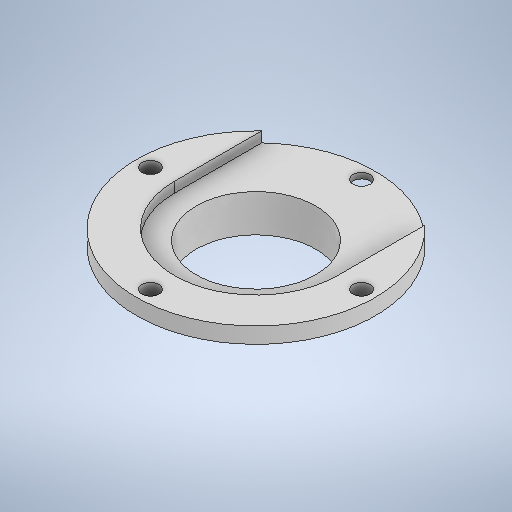
# Autodesk Inventor part: LoadCellMount
Saved by Autodesk Inventor 2025.2 (Build 292293000, 293)
## iProperties
Created: 2025-07-29
Part Number: LoadCellMount
Material: Generic
Document SubType Name: Modeling
Designer: Simon
Density: 1 g/cm^3
Appearance: Default
Author: Simon
Autodesk Inventor part; units mm, degrees
ref_plane "YZ Plane" through (0, 0, 0) normal (1, 0, 0) x (0, 1, 0)
ref_plane "XZ Plane" through (0, 0, 0) normal (0, 1, 0) x (-1, 0, 0)
ref_plane "XY Plane" through (0, 0, 0) normal (0, 0, 1) x (1, 0, 0)
sketch "Sketch1" plane through (0, 0, 0) normal (0, 1, 0) x (-1, 0, 0)
  circle A0 centre (0, 0) radius 30
  circle A1 centre (0, 0) radius 22.5
  circle A2 centre (0, 0) radius 26.5
  circle A3 centre (0, 26.5) radius 2.15
  circle A4 centre (-26.5, 0) radius 2.15
  circle A5 centre (0, -26.5) radius 2.15
  circle A6 centre (26.5, 0) radius 2.15
  dimension "d3" = 53
  dimension "d0" = 60
  dimension "d1" = 45
  dimension "d4" = 4.3
  dimension "d7" = 360
  constraints: 6 centre point, 3 coincident, 1 vertical alignment, 11 other
  measures "d0" diameter of A0
  measures "d1" diameter of A1
  measures "d4" diameter of A3
extrude "Extrusion1" add sketch "Sketch1" against normal blind 4 contours A0 | A1 | A6 A2 A5 A4 A3
sketch "Sketch2" plane through (0, 0, 0) normal (0, 1, 0) x (1, 0, 0)
  circle A0 centre (0, 0) radius 20.5
  line L0 (-20.5, 0) -> (-20.5, 21.9032)
  circle A1 centre (0, 0) radius 30 projected
  line L1 (20.5, 0) -> (20.5, 21.9032)
  circle A2 centre (0, 0) radius 30
  dimension "d11" = 41
  constraints: 4 end point, 4 point on circle, 2 centre point, 2 coincident, 1 concentric, 1 parallel, 1 tangent, 1 vertical
  measures "d11" diameter of A0
extrude "Extrusion2" cut sketch "Sketch2" against normal blind 2.6 contours A0 | A0 L0 A1 L1 picked at (-0.8237, 26.6681)
sketch "Sketch3" plane through (0, -4, 0) normal (0, -1, 0) x (1, 0, 0)
  circle A0 centre (0, 0) radius 15
  dimension "d14" = 30
  constraints: 1 centre point, 1 coincident
  measures "d14" diameter of A0
extrude "Extrusion3" cut sketch "Sketch3" against normal through all
sketch "Sketch4" plane through (0, -4, 0) normal (0, -1, 0) x (1, 0, 0)
  circle A0 centre (0, 0) radius 15
  circle A1 centre (0, 0) radius 17.5
  dimension "d17" = 30
  dimension "d18" = 35
  constraints: 2 centre point, 2 coincident
  measures "d17" diameter of A0
  measures "d18" diameter of A1
extrude "Extrusion4" add sketch "Sketch4" along normal blind 8
body "Solid1"
